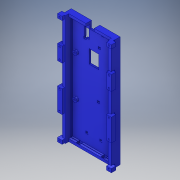
# Autodesk Inventor part: BODY_BOTTOM_2
Saved by Autodesk Inventor 2017 (Build 210142000, 142)
## iProperties
Created: 2018-07-28
Part Number: BODY_BOTTOM_2
Material: Generic
Document SubType Name: Modeling
Designer: Alexander Miller
Density: 1 g/cm^3
Appearance: Blue - Wall Paint - Glossy
Author: Alexander Miller
Autodesk Inventor part; units mm, degrees
ref_plane "YZ Plane" through (0, 0, 0) normal (1, 0, 0) x (0, 1, 0)
ref_plane "XZ Plane" through (0, 0, 0) normal (0, 1, 0) x (-1, 0, 0)
ref_plane "XY Plane" through (0, 0, 0) normal (0, 0, 1) x (1, 0, 0)
sketch "Sketch1" plane through (0, 0, 0) normal (0, 0, 1) x (1, 0, 0)
  line L0 (-34.885, -79.35) -> (34.885, -79.35)
  line L1 (34.885, -79.35) -> (34.885, 79.35)
  line L2 (34.885, 79.35) -> (-34.885, 79.35)
  line L3 (-34.885, 79.35) -> (-34.885, -79.35)
  point P0 (0, 0)
  point P1 (0, 79.35)
  point P2 (34.885, 0)
  point P3 (0, -79.35)
  dimension "d0" = 158.7
  dimension "d1" = 69.77
  constraints: 8 end point, 3 midpoint, 2 parallel, 1 horizontal, 1 horizontal alignment, 1 perpendicular, 1 vertical alignment
  measures "d0" distance of L0.end L1.end
  measures "d1" distance of L1.end L2.end
extrude "Extrusion1" add sketch "Sketch1" along normal blind 5
sketch "Sketch3" plane through (0, 0, 5) normal (0, 0, 1) x (1, 0, 0)
  line L0 (-34.885, 79.35) -> (-30.5, 79.35)
  line L1 (-30.5, 79.35) -> (-30.5, -79.35)
  line L2 (-30.5, -79.35) -> (-34.885, -79.35)
  line L3 (-34.885, -79.35) -> (-34.885, 79.35)
  line L4 (30.5, 79.35) -> (34.885, 79.35)
  line L5 (34.885, 79.35) -> (34.885, -79.35)
  line L6 (34.885, -79.35) -> (30.5, -79.35)
  line L7 (30.5, -79.35) -> (30.5, 79.35)
  line L8 (34.885, 79.35) -> (-34.885, 79.35) projected
  line L9 (-34.885, 79.35) -> (-34.885, -79.35) projected
  line L10 (-34.885, -79.35) -> (34.885, -79.35) projected
  line L11 (34.885, -79.35) -> (34.885, 79.35) projected
  point P0 (0, 0)
  dimension "d14" = 4.385
  constraints: 16 end point, 7 collinear, 4 parallel, 2 horizontal, 2 perpendicular
  measures "d14" distance of L0.start L0.end
extrude "Extrusion3" add sketch "Sketch3" along normal blind 7.74 contours L0 L1 L2 L3 | L4 L5 L6 L7
sketch "Sketch4" plane through (0, 0, 12.74) normal (0, 0, 1) x (1, 0, 0)
  line L0 (31.885, -74.1) -> (38.635, -74.1)
  line L1 (38.635, -74.1) -> (38.635, -79.35)
  line L2 (38.635, -79.35) -> (31.885, -79.35)
  line L3 (31.885, -79.35) -> (31.885, -74.1)
  line L4 (30.5, 79.35) -> (30.5, -79.35) projected
  line L5 (30.5, -79.35) -> (34.885, -79.35) projected
  line L6 (31.885, -37.15) -> (38.635, -37.15)
  line L7 (38.635, -37.15) -> (38.635, -42.4)
  line L8 (38.635, -42.4) -> (31.885, -42.4)
  line L9 (31.885, -42.4) -> (31.885, -37.15)
  line L10 (31.885, -10.35) -> (38.635, -10.35)
  line L11 (38.635, -10.35) -> (38.635, -15.6)
  line L12 (38.635, -15.6) -> (31.885, -15.6)
  line L13 (31.885, -15.6) -> (31.885, -10.35)
  line L14 (31.885, 26.6) -> (38.635, 26.6)
  line L15 (38.635, 26.6) -> (38.635, 21.35)
  line L16 (38.635, 21.35) -> (31.885, 21.35)
  line L17 (31.885, 21.35) -> (31.885, 26.6)
  line L18 (31.885, 42.4) -> (38.635, 42.4)
  line L19 (38.635, 42.4) -> (38.635, 37.15)
  line L20 (38.635, 37.15) -> (31.885, 37.15)
  line L21 (31.885, 37.15) -> (31.885, 42.4)
  line L22 (31.885, 79.35) -> (38.635, 79.35)
  line L23 (38.635, 79.35) -> (38.635, 74.1)
  line L24 (38.635, 74.1) -> (31.885, 74.1)
  line L25 (31.885, 74.1) -> (31.885, 79.35)
  line L26 (34.885, 79.35) -> (30.5, 79.35) projected
  line L27 (41.26, 21.35) -> (29.26, 21.35) construction
  line L28 (29.26, 21.35) -> (29.26, -10.35) construction
  line L29 (29.26, -10.35) -> (41.26, -10.35) construction
  line L30 (41.26, -10.35) -> (41.26, 21.35) construction
  circle A0 centre (35.26, 0) radius 6 construction
  line L31 (0, -111.09) -> (0, 111.09) projected
  line L32 (-31.885, -74.1) -> (-38.635, -74.1)
  line L33 (-38.635, -74.1) -> (-38.635, -79.35)
  line L34 (-38.635, -79.35) -> (-31.885, -79.35)
  line L35 (-31.885, -79.35) -> (-31.885, -74.1)
  line L36 (-30.5, -79.35) -> (-34.885, -79.35)
  line L37 (-31.885, -37.15) -> (-38.635, -37.15)
  line L38 (-38.635, -37.15) -> (-38.635, -42.4)
  line L39 (-38.635, -42.4) -> (-31.885, -42.4)
  line L40 (-31.885, -42.4) -> (-31.885, -37.15)
  line L41 (-31.885, -10.35) -> (-38.635, -10.35)
  line L42 (-38.635, -10.35) -> (-38.635, -15.6)
  line L43 (-38.635, -15.6) -> (-31.885, -15.6)
  line L44 (-31.885, -15.6) -> (-31.885, -10.35)
  line L45 (-31.885, 26.6) -> (-38.635, 26.6)
  line L46 (-38.635, 26.6) -> (-38.635, 21.35)
  line L47 (-38.635, 21.35) -> (-31.885, 21.35)
  line L48 (-31.885, 21.35) -> (-31.885, 26.6)
  line L49 (-31.885, 42.4) -> (-38.635, 42.4)
  line L50 (-38.635, 42.4) -> (-38.635, 37.15)
  line L51 (-38.635, 37.15) -> (-31.885, 37.15)
  line L52 (-31.885, 37.15) -> (-31.885, 42.4)
  line L53 (-31.885, 79.35) -> (-38.635, 79.35)
  line L54 (-38.635, 79.35) -> (-38.635, 74.1)
  line L55 (-38.635, 74.1) -> (-31.885, 74.1)
  line L56 (-31.885, 74.1) -> (-31.885, 79.35)
  line L57 (-34.885, 79.35) -> (-30.5, 79.35)
  line L58 (-41.26, 21.35) -> (-29.26, 21.35) construction
  line L59 (-29.26, -10.35) -> (-41.26, -10.35) construction
  line L60 (-41.26, -10.35) -> (-41.26, 21.35) construction
  circle A1 centre (-35.26, 0) radius 6 construction
  line L61 (29.26, 17) -> (41.26, 17) construction
  line L62 (41.26, 17) -> (41.26, -6) construction
  line L63 (41.26, -6) -> (29.26, -6) construction
  line L64 (29.26, -6) -> (29.26, 17) construction
  line L65 (-38.635, -37.15) -> (-31.885, -37.15)
  line L66 (-31.885, -37.15) -> (-31.885, -15.6)
  line L67 (-31.885, -15.6) -> (-38.635, -15.6)
  line L68 (-38.635, -15.6) -> (-38.635, -37.15)
  line L69 (31.885, -37.15) -> (38.635, -37.15)
  line L70 (38.635, -37.15) -> (38.635, -15.6)
  line L71 (38.635, -15.6) -> (31.885, -15.6)
  line L72 (31.885, -15.6) -> (31.885, -37.15)
  line L73 (-38.635, 26.6) -> (-31.885, 26.6)
  line L74 (-31.885, 26.6) -> (-31.885, 37.15)
  line L75 (-31.885, 37.15) -> (-38.635, 37.15)
  line L76 (-38.635, 37.15) -> (-38.635, 26.6)
  line L77 (31.885, 26.6) -> (38.635, 26.6)
  line L78 (38.635, 26.6) -> (38.635, 37.15)
  line L79 (38.635, 37.15) -> (31.885, 37.15)
  line L80 (31.885, 37.15) -> (31.885, 26.6)
  line L81 (-31.885, 74.1) -> (-30.5, 74.1)
  line L82 (-30.5, 74.1) -> (-30.5, 79.35)
  line L83 (-30.5, 79.35) -> (-31.885, 79.35)
  line L84 (-31.885, 79.35) -> (-31.885, 74.1)
  line L85 (-31.885, 42.4) -> (-30.5, 42.4)
  line L86 (-30.5, 42.4) -> (-30.5, 21.35)
  line L87 (-30.5, 21.35) -> (-31.885, 21.35)
  line L88 (-31.885, 21.35) -> (-31.885, 42.4)
  line L89 (-31.885, -10.35) -> (-30.5, -10.35)
  line L90 (-30.5, -10.35) -> (-30.5, -42.4)
  line L91 (-30.5, -42.4) -> (-31.885, -42.4)
  line L92 (-31.885, -42.4) -> (-31.885, -10.35)
  line L93 (-31.885, -74.1) -> (-30.5, -74.1)
  line L94 (-30.5, -74.1) -> (-30.5, -79.35)
  line L95 (-30.5, -79.35) -> (-31.885, -79.35)
  line L96 (-31.885, -79.35) -> (-31.885, -74.1)
  line L97 (30.5, 79.35) -> (31.885, 79.35)
  line L98 (31.885, 79.35) -> (31.885, 74.1)
  line L99 (31.885, 74.1) -> (30.5, 74.1)
  line L100 (30.5, 74.1) -> (30.5, 79.35)
  line L101 (30.5, 42.4) -> (31.885, 42.4)
  line L102 (31.885, 42.4) -> (31.885, 21.35)
  line L103 (31.885, 21.35) -> (30.5, 21.35)
  line L104 (30.5, 21.35) -> (30.5, 42.4)
  line L105 (30.5, -10.35) -> (31.885, -10.35)
  line L106 (31.885, -10.35) -> (31.885, -42.4)
  line L107 (31.885, -42.4) -> (30.5, -42.4)
  line L108 (30.5, -42.4) -> (30.5, -10.35)
  line L109 (30.5, -74.1) -> (31.885, -74.1)
  line L110 (31.885, -74.1) -> (31.885, -79.35)
  line L111 (31.885, -79.35) -> (30.5, -79.35)
  line L112 (30.5, -79.35) -> (30.5, -74.1)
  line L113 (-30.5, -79.35) -> (-30.5, 79.35) projected
  line L114 (-34.885, -79.35) -> (-30.5, -79.35) projected
  point P0 (0, 0)
  point P1 (35.26, 74.1)
  point P2 (35.26, 42.4)
  point P3 (35.26, 37.15)
  point P4 (35.26, 26.6)
  point P5 (35.26, 21.35)
  point P6 (35.26, -10.35)
  point P7 (35.26, -15.6)
  point P8 (35.26, -37.15)
  point P9 (35.26, -42.4)
  point P10 (35.26, -74.1)
  point P11 (35.26, 21.35)
  point P12 (-35.26, 74.1)
  point P13 (-35.26, 42.4)
  point P14 (-35.26, 37.15)
  point P15 (-35.26, 26.6)
  point P16 (-35.26, 21.35)
  point P17 (-35.26, -10.35)
  point P18 (-35.26, -15.6)
  point P19 (-35.26, -37.15)
  point P20 (-35.26, -42.4)
  point P21 (-35.26, -74.1)
  point P22 (-35.26, 21.35)
  point P23 (29.26, 5.5)
  point P24 (29.26, 5.5)
  dimension "d17" = 6.75
  dimension "d18" = 1.385
  dimension "d19" = 5.25
  dimension "d40" = 31.7
  dimension "d41" = 31.7
  dimension "d42" = 31.7
  dimension "d43" = 12
  dimension "d44" = 23
  constraints: 218 end point, 44 symmetric about line, 40 parallel, 34 collinear, 20 horizontal, 20 perpendicular, 13 midpoint, 10 equal length, 5 vertical alignment, 3 tangent, 2 centre point, 2 coincident, 1 horizontal alignment, 1 other
  measures "d17" distance of L0.start L0.end
  measures "d18" distance between parallel lines of L3 L4
  measures "d19" distance of L0.end L1.end
  measures "d40" distance between parallel lines of L0 L8
  measures "d41" distance between parallel lines of L10 L16
  measures "d42" distance between parallel lines of L18 L24
  measures "d43" distance of L27.start L27.end
  measures "d44" distance between parallel lines of L63 L61
extrude "Extrusion4" add sketch "Sketch4" along normal blind 3.5 and the other way blind 5 contours L0 L1 L2 L3 | L9 L6 L7 L8 | L10 L11 L12 L13 | L72 L12 L70 L6 | L17 L14 L15 L16 | L18 L19 L20 L21 | L80 L20 L78 L14 | L25 L22 L23 L24 | L35 L34 L33 L32 | L39 L38 L37 L40 | L44 L43 L42 L41 | L37 L68 L43 L66 | L47 L46 L45 L48 | L52 L51 L50 L49 | L45 L76 L51 L74 | L55 L54 L53 L56
sketch "Sketch7" plane through (0, 0, 7.74) normal (0, 0, -1) x (-1, 0, 0)
  line L0 (-33.085, -78.85) -> (-37.435, -78.85)
  line L1 (-37.435, -78.85) -> (-37.435, -74.5)
  line L2 (-37.435, -74.5) -> (-33.085, -74.5)
  line L3 (-33.085, -74.5) -> (-33.085, -78.85)
  line L4 (-38.635, -74.1) -> (-38.635, -79.35) projected
  line L5 (-31.885, -79.35) -> (-38.635, -79.35) projected
  line L6 (-33.085, -37.65) -> (-37.435, -37.65)
  line L7 (-37.435, -37.65) -> (-37.435, -42)
  line L8 (-37.435, -42) -> (-33.085, -42)
  line L9 (-33.085, -42) -> (-33.085, -37.65)
  line L10 (-33.085, -10.75) -> (-37.435, -10.75)
  line L11 (-37.435, -10.75) -> (-37.435, -15.1)
  line L12 (-37.435, -15.1) -> (-33.085, -15.1)
  line L13 (-33.085, -15.1) -> (-33.085, -10.75)
  line L14 (-33.085, 26.1) -> (-37.435, 26.1)
  line L15 (-37.435, 26.1) -> (-37.435, 21.75)
  line L16 (-37.435, 21.75) -> (-33.085, 21.75)
  line L17 (-33.085, 21.75) -> (-33.085, 26.1)
  line L18 (-33.085, 42) -> (-37.435, 42)
  line L19 (-37.435, 42) -> (-37.435, 37.65)
  line L20 (-37.435, 37.65) -> (-33.085, 37.65)
  line L21 (-33.085, 37.65) -> (-33.085, 42)
  line L22 (-33.085, 78.85) -> (-37.435, 78.85)
  line L23 (-37.435, 78.85) -> (-37.435, 74.5)
  line L24 (-37.435, 74.5) -> (-33.085, 74.5)
  line L25 (-33.085, 74.5) -> (-33.085, 78.85)
  line L26 (-38.635, 79.35) -> (-38.635, 74.1) projected
  line L27 (0, -111.09) -> (0, 111.09) projected
  line L28 (33.085, -78.85) -> (37.435, -78.85)
  line L29 (37.435, -78.85) -> (37.435, -74.5)
  line L30 (37.435, -74.5) -> (33.085, -74.5)
  line L31 (33.085, -74.5) -> (33.085, -78.85)
  line L32 (33.085, -37.65) -> (37.435, -37.65)
  line L33 (37.435, -37.65) -> (37.435, -42)
  line L34 (37.435, -42) -> (33.085, -42)
  line L35 (33.085, -42) -> (33.085, -37.65)
  line L36 (33.085, -10.75) -> (37.435, -10.75)
  line L37 (37.435, -10.75) -> (37.435, -15.1)
  line L38 (37.435, -15.1) -> (33.085, -15.1)
  line L39 (33.085, -15.1) -> (33.085, -10.75)
  line L40 (33.085, 26.1) -> (37.435, 26.1)
  line L41 (37.435, 26.1) -> (37.435, 21.75)
  line L42 (37.435, 21.75) -> (33.085, 21.75)
  line L43 (33.085, 21.75) -> (33.085, 26.1)
  line L44 (33.085, 42) -> (37.435, 42)
  line L45 (37.435, 42) -> (37.435, 37.65)
  line L46 (37.435, 37.65) -> (33.085, 37.65)
  line L47 (33.085, 37.65) -> (33.085, 42)
  line L48 (33.085, 78.85) -> (37.435, 78.85)
  line L49 (37.435, 78.85) -> (37.435, 74.5)
  line L50 (37.435, 74.5) -> (33.085, 74.5)
  line L51 (33.085, 74.5) -> (33.085, 78.85)
  line L52 (-38.635, -79.35) -> (-34.885, -79.35) projected
  line L53 (-34.885, -74.1) -> (-34.885, -79.35) projected
  line L54 (-38.635, -79.35) -> (-34.885, -79.35)
  line L55 (-34.885, -79.35) -> (-34.885, -74.1)
  line L56 (-34.885, -74.1) -> (-38.635, -74.1)
  line L57 (-38.635, -74.1) -> (-38.635, -79.35)
  line L58 (-34.885, 79.35) -> (-38.635, 79.35) projected
  line L59 (-38.635, -42.4) -> (-34.885, -42.4) projected
  line L60 (-34.885, -10.35) -> (-38.635, -10.35) projected
  line L61 (-38.635, 21.35) -> (-34.885, 21.35) projected
  line L62 (-34.885, 42.4) -> (-38.635, 42.4) projected
  line L63 (-38.635, -42.4) -> (-34.885, -42.4)
  line L64 (-34.885, -42.4) -> (-34.885, -10.35)
  line L65 (-34.885, -10.35) -> (-38.635, -10.35)
  line L66 (-38.635, -10.35) -> (-38.635, -42.4)
  line L67 (-38.635, 21.35) -> (-38.635, 42.4) projected
  line L68 (-38.635, 21.35) -> (-34.885, 21.35)
  line L69 (-34.885, 21.35) -> (-34.885, 42.4)
  line L70 (-34.885, 42.4) -> (-38.635, 42.4)
  line L71 (-38.635, 42.4) -> (-38.635, 21.35)
  line L72 (-31.885, 74.1) -> (-38.635, 74.1) projected
  line L73 (-34.885, -79.35) -> (-34.885, 79.35) projected
  line L74 (-38.635, 74.1) -> (-34.885, 74.1)
  line L75 (-34.885, 74.1) -> (-34.885, 79.35)
  line L76 (-34.885, 79.35) -> (-38.635, 79.35)
  line L77 (-38.635, 79.35) -> (-38.635, 74.1)
  line L78 (38.635, -74.1) -> (38.635, -79.35) projected
  line L79 (34.885, 79.35) -> (34.885, -79.35) projected
  line L80 (38.635, -74.1) -> (34.885, -74.1)
  line L81 (34.885, -74.1) -> (34.885, -79.35)
  line L82 (34.885, -79.35) -> (38.635, -79.35)
  line L83 (38.635, -79.35) -> (38.635, -74.1)
  line L84 (38.635, -42.4) -> (38.635, -10.35) projected
  line L85 (34.885, -42.4) -> (34.885, -10.35) projected
  line L86 (38.635, -10.35) -> (34.885, -10.35)
  line L87 (34.885, -10.35) -> (34.885, -42.4)
  line L88 (34.885, -42.4) -> (38.635, -42.4)
  line L89 (38.635, -42.4) -> (38.635, -10.35)
  line L90 (38.635, 21.35) -> (38.635, 42.4) projected
  line L91 (38.635, 42.4) -> (34.885, 42.4)
  line L92 (34.885, 42.4) -> (34.885, 21.35)
  line L93 (34.885, 21.35) -> (38.635, 21.35)
  line L94 (38.635, 21.35) -> (38.635, 42.4)
  line L95 (38.635, 79.35) -> (38.635, 74.1) projected
  line L96 (38.635, 79.35) -> (34.885, 79.35)
  line L97 (34.885, 79.35) -> (34.885, 74.1)
  line L98 (34.885, 74.1) -> (38.635, 74.1)
  line L99 (38.635, 74.1) -> (38.635, 79.35)
  point P0 (0, 0)
  point P1 (-37.435, -76.675)
  point P2 (-35.26, -79.35)
  point P3 (-35.26, -78.85)
  point P4 (-35.26, -74.5)
  point P5 (-35.26, -42)
  point P6 (-35.26, -37.65)
  point P7 (-35.26, -15.1)
  point P8 (-35.26, -10.75)
  point P9 (-35.26, 21.75)
  point P10 (-35.26, 26.1)
  point P11 (-35.26, 37.65)
  point P12 (-35.26, 42)
  point P13 (-35.26, 74.5)
  point P14 (-37.435, -39.825)
  point P15 (-38.635, -39.825)
  point P16 (-37.435, -12.925)
  point P17 (-38.635, -12.925)
  point P18 (-37.435, 23.925)
  point P19 (-38.635, 23.925)
  point P20 (-37.435, 39.825)
  point P21 (-38.635, 39.825)
  point P22 (-37.435, 76.675)
  point P23 (-38.635, 76.725)
  point P24 (37.435, -76.675)
  point P25 (31.885, -79.35)
  point P26 (35.26, -79.35)
  point P27 (35.26, -78.85)
  point P28 (35.26, -74.5)
  point P29 (35.26, -42)
  point P30 (35.26, -37.65)
  point P31 (35.26, -15.1)
  point P32 (35.26, -10.75)
  point P33 (35.26, 21.75)
  point P34 (35.26, 26.1)
  point P35 (35.26, 37.65)
  point P36 (35.26, 42)
  point P37 (35.26, 74.5)
  point P38 (37.435, -39.825)
  point P39 (37.435, -12.925)
  point P40 (37.435, 23.925)
  point P41 (37.435, 39.825)
  point P42 (37.435, 76.725)
  dimension "d45" = 4.35
  dimension "d142" = 2.675
  dimension "d143" = 2.675
  dimension "d144" = 2.575
  dimension "d145" = 2.575
  dimension "d146" = 2.575
  dimension "d147" = 2.575
  constraints: 160 end point, 42 symmetric about line, 28 parallel, 19 midpoint, 14 horizontal, 14 perpendicular, 11 equal length, 6 vertical alignment, 4 horizontal alignment, 4 point on line
  measures "d45" distance of L0.end L1.end
  measures "d142" distance from line of point (-37.435, -76.675) L5
  measures "d143" distance from line of point (-37.435, 76.675) L58
  measures "d144" distance from line of L59 point (-37.435, -39.825)
  measures "d145" distance from line of point (-37.435, -12.925) L60
  measures "d146" distance from line of L61 point (-37.435, 23.925)
  measures "d147" distance from line of point (-37.435, 39.825) L62
extrude "Extrusion7" cut sketch "Sketch7" against normal blind 2.075
sketch "Sketch8" plane through (0, 0, 16.24) normal (0, 0, 1) x (1, 0, 0)
  circle A0 centre (35.26, -76.675) radius 1.175
  line L0 (31.885, -74.1) -> (31.885, -79.35) projected
  line L1 (38.635, -74.1) -> (31.885, -74.1) projected
  circle A1 centre (35.26, -39.825) radius 1.175
  circle A2 centre (35.26, -12.925) radius 1.175
  circle A3 centre (35.26, 23.925) radius 1.175
  circle A4 centre (35.26, 39.825) radius 1.175
  circle A5 centre (35.26, 76.675) radius 1.175
  line L2 (31.885, 79.35) -> (31.885, 74.1) projected
  line L3 (0, -111.09) -> (0, 111.09) projected
  circle A6 centre (-35.26, -76.675) radius 1.175
  circle A7 centre (-35.26, -39.825) radius 1.175
  circle A8 centre (-35.26, -12.925) radius 1.175
  circle A9 centre (-35.26, 23.925) radius 1.175
  circle A10 centre (-35.26, 39.825) radius 1.175
  circle A11 centre (-35.26, 76.675) radius 1.175
  line L4 (31.885, -79.35) -> (38.635, -79.35) projected
  line L5 (31.885, -42.4) -> (38.635, -42.4) projected
  line L6 (38.635, -10.35) -> (31.885, -10.35) projected
  line L7 (31.885, 21.35) -> (38.635, 21.35) projected
  line L8 (38.635, 42.4) -> (31.885, 42.4) projected
  line L9 (38.635, 79.35) -> (31.885, 79.35) projected
  point P0 (0, 0)
  point P1 (31.885, -76.725)
  point P2 (35.26, -74.1)
  point P3 (31.885, 76.725)
  point P4 (31.885, 39.825)
  point P5 (31.885, 23.925)
  point P6 (31.885, -12.925)
  point P7 (31.885, -39.825)
  point P8 (-35.26, -74.1)
  point P9 (-38.635, -74.1)
  dimension "d48" = 2.35
  dimension "d148" = 2.675
  dimension "d149" = 2.575
  dimension "d150" = 2.575
  dimension "d151" = 2.575
  dimension "d152" = 2.575
  dimension "d153" = 2.675
  constraints: 12 centre point, 8 symmetric about line, 6 vertical alignment, 5 equal radius, 4 horizontal alignment, 3 midpoint, 6 other
  measures "d48" diameter of A0
  measures "d148" distance from line of L4 A0.centre
  measures "d149" distance from line of L5 A1.centre
  measures "d150" distance from line of L6 A2.centre
  measures "d151" distance from line of L7 A3.centre
  measures "d152" distance from line of A4.centre L8
  measures "d153" distance from line of L9 A5.centre
extrude "Extrusion8" cut sketch "Sketch8" against normal up to surface (6.425 mm away)
sketch "Sketch9" plane through (0, 0, 5) normal (0, 0, 1) x (1, 0, 0)
  circle A0 centre (-25, 31.875) radius 1.25
  line L0 (30.5, 79.35) -> (-30.5, 79.35) projected
  line L1 (0, -111.09) -> (0, 111.09) projected
  line L2 (-48.839, 0) -> (48.839, 0) projected
  circle A1 centre (-25, -26.375) radius 1.25
  circle A2 centre (25, 31.875) radius 1.25
  circle A3 centre (25, -26.375) radius 1.25
  point P0 (0, 0)
  dimension "d52" = 31.875
  dimension "d53" = 25
  dimension "d54" = 2.5
  dimension "d57" = 58.25
  constraints: 4 centre point, 2 symmetric about line, 1 equal radius, 1 vertical alignment, 2 other
  measures "d52" vertical distance of point (0, 0) A0.centre
  measures "d53" horizontal distance of A0.centre point (0, 0)
  measures "d54" diameter of A0
  measures "d57" distance of A1.centre A0.centre
extrude "Extrusion9" cut sketch "Sketch9" against normal through all
sketch "Sketch10" plane through (0, 0, 5) normal (0, 0, 1) x (1, 0, 0)
  line L0 (30.25, -75.25) -> (-30.25, -75.25)
  line L1 (-30.25, -75.25) -> (-30.25, 75.25)
  line L2 (-30.25, 75.25) -> (30.25, 75.25)
  line L3 (30.25, 75.25) -> (30.25, -75.25)
  circle A0 centre (25, -26.375) radius 3.25
  circle A1 centre (-25, -26.375) radius 3.25
  circle A2 centre (25, 31.875) radius 3.25
  circle A3 centre (-25, 31.875) radius 3.25
  circle A4 centre (25, -26.375) radius 1.25 projected
  circle A5 centre (-25, -26.375) radius 1.25 projected
  circle A6 centre (-25, 31.875) radius 1.25 projected
  circle A7 centre (25, 31.875) radius 1.25 projected
  point P0 (0, 0)
  point P1 (-30.25, 0)
  point P2 (0, -75.25)
  dimension "d58" = 150.5
  dimension "d59" = 60.5
  dimension "d61" = 2
  constraints: 8 end point, 4 centre point, 4 concentric, 3 equal radius, 2 midpoint, 2 parallel, 1 horizontal, 1 horizontal alignment, 1 perpendicular, 1 vertical alignment
  measures "d58" distance of L0.end L1.end
  measures "d59" distance of L0.start L0.end
  measures "d61" radial gap between concentric circles of A0 A4
extrude "Extrusion10" cut sketch "Sketch10" against normal blind 2.5 contours L0 L1 L2 L3
sketch "Sketch12" plane through (0, 0, 5) normal (0, 0, 1) x (1, 0, 0)
  line L0 (-6, 79.35) -> (6, 79.35)
  line L1 (6, 79.35) -> (6, 70)
  line L2 (6, 70) -> (-6, 70)
  line L3 (-6, 70) -> (-6, 79.35)
  line L4 (30.5, 79.35) -> (-30.5, 79.35) projected
  point P0 (0, 0)
  point P1 (0, 79.35)
  point P2 (0, 79.35)
  dimension "d68" = 9.35
  dimension "d69" = 12
  constraints: 8 end point, 2 midpoint, 2 parallel, 1 coincident, 1 collinear, 1 horizontal, 1 perpendicular
  measures "d68" distance of L2.end L0.start
  measures "d69" distance of L1.end L2.end
extrude "Extrusion12" cut sketch "Sketch12" against normal through all
sketch "Sketch13" plane through (0, 0, 0) normal (0, 0, -1) x (-1, 0, 0)
  line L0 (-7, 45.14) -> (7, 45.14)
  line L1 (7, 45.14) -> (7, 38.54)
  line L2 (7, 38.54) -> (-7, 38.54)
  line L3 (-7, 38.54) -> (-7, 45.14)
  line L4 (-7, 38.79) -> (7, 38.79)
  line L5 (7, 38.79) -> (7, 32.19)
  line L6 (7, 32.19) -> (-7, 32.19)
  line L7 (-7, 32.19) -> (-7, 38.79)
  line L8 (-7, 32.44) -> (7, 32.44)
  line L9 (7, 32.44) -> (7, 25.84)
  line L10 (7, 25.84) -> (-7, 25.84)
  line L11 (-7, 25.84) -> (-7, 32.44)
  line L12 (-13.791, 74.201) -> (-10.791, 74.201)
  line L13 (-10.791, 74.201) -> (-10.791, 71.201)
  line L14 (-10.791, 71.201) -> (-13.791, 71.201)
  line L15 (-13.791, 71.201) -> (-13.791, 74.201)
  line L16 (-9.244, 54.465) -> (-6.244, 54.465)
  line L17 (-6.244, 54.465) -> (-6.244, 51.465)
  line L18 (-6.244, 51.465) -> (-9.244, 51.465)
  line L19 (-9.244, 51.465) -> (-9.244, 54.465)
  line L20 (11.279, 56.853) -> (14.279, 56.853)
  line L21 (14.279, 56.853) -> (14.279, 53.853)
  line L22 (14.279, 53.853) -> (11.279, 53.853)
  line L23 (11.279, 53.853) -> (11.279, 56.853)
  line L24 (-8.051, -13.023) -> (-5.051, -13.023)
  line L25 (-5.051, -13.023) -> (-5.051, -16.023)
  line L26 (-5.051, -16.023) -> (-8.051, -16.023)
  line L27 (-8.051, -16.023) -> (-8.051, -13.023)
  line L28 (-11.53, -59.149) -> (-8.53, -59.149)
  line L29 (-8.53, -59.149) -> (-8.53, -62.149)
  line L30 (-8.53, -62.149) -> (-11.53, -62.149)
  line L31 (-11.53, -62.149) -> (-11.53, -59.149)
  line L32 (8.485, -59.149) -> (11.485, -59.149)
  line L33 (11.485, -59.149) -> (11.485, -62.149)
  line L34 (11.485, -62.149) -> (8.485, -62.149)
  line L35 (8.485, -62.149) -> (8.485, -59.149)
  line L36 (-13.791, 72.296) -> (-10.791, 72.296)
  line L37 (-10.791, 72.296) -> (-10.791, 69.296)
  line L38 (-10.791, 69.296) -> (-13.791, 69.296)
  line L39 (-13.791, 69.296) -> (-13.791, 72.296)
  line L40 (6.637, 69.673) -> (13.637, 69.673)
  line L41 (13.637, 69.673) -> (13.637, 62.673)
  line L42 (13.637, 62.673) -> (6.637, 62.673)
  line L43 (6.637, 62.673) -> (6.637, 69.673)
  line L44 (13.637, 63.399) -> (6.637, 63.399)
  line L45 (6.637, 63.399) -> (6.637, 56.399)
  line L46 (6.637, 56.399) -> (13.637, 56.399)
  line L47 (13.637, 56.399) -> (13.637, 63.399)
  point P0 (0, 0)
  point P1 (0, 38.54)
  point P2 (7, 41.84)
  point P3 (0, 38.79)
  point P4 (0, 32.19)
  point P5 (0, 32.44)
  point P6 (7, 35.49)
  point P7 (7, 29.14)
  point P8 (-10.791, 72.701)
  point P9 (-12.291, 71.201)
  point P10 (-12.291, 72.296)
  point P11 (-10.791, 70.796)
  point P12 (-6.244, 52.965)
  point P13 (-7.744, 51.465)
  point P14 (12.779, 53.853)
  point P15 (11.279, 55.353)
  point P16 (-6.551, -13.023)
  point P17 (-5.051, -14.523)
  point P18 (-10.03, -59.149)
  point P19 (-11.53, -60.649)
  point P20 (9.985, -59.149)
  point P21 (11.485, -60.649)
  point P22 (13.637, 66.173)
  point P23 (10.137, 62.673)
  point P24 (6.637, 59.899)
  point P25 (10.137, 56.399)
  point P26 (10.137, 63.399)
  dimension "d72" = 41.84
  dimension "d73" = 14
  dimension "d74" = 6.6
  dimension "d77" = 35.49
  dimension "d78" = 29.14
  dimension "d79" = 12.291
  dimension "d80" = 72.701
  dimension "d81" = 3
  dimension "d83" = 70.796
  dimension "d84" = 7.744
  dimension "d85" = 52.965
  dimension "d86" = 12.779
  dimension "d87" = 55.353
  dimension "d88" = 6.551
  dimension "d89" = 14.523
  dimension "d90" = 10.03
  dimension "d91" = 60.649
  dimension "d92" = 9.985
  dimension "d93" = 60.649
  dimension "d133" = 10.137
  dimension "d134" = 66.173
  dimension "d135" = 7
  dimension "d136" = 7
  dimension "d138" = 59.899
  constraints: 96 end point, 26 midpoint, 24 parallel, 19 equal length, 12 horizontal, 12 perpendicular, 5 vertical alignment
  measures "d72" vertical distance of point (7, 41.84) point (0, 0)
  measures "d73" distance of L0.start L0.end
  measures "d74" distance of L2.end L0.start
  measures "d77" vertical distance of point (7, 35.49) point (0, 0)
  measures "d78" vertical distance of point (7, 29.14) point (0, 0)
  measures "d79" horizontal distance of point (-12.291, 71.201) point (0, 0)
  measures "d80" vertical distance of point (0, 0) point (-10.791, 72.701)
  measures "d81" distance of L14.end L12.start
  measures "d83" vertical distance of point (0, 0) point (-10.791, 70.796)
  measures "d84" horizontal distance of point (-7.744, 51.465) point (0, 0)
  measures "d85" vertical distance of point (-6.244, 52.965) point (0, 0)
  measures "d86" horizontal distance of point (0, 0) point (12.779, 53.853)
  measures "d87" vertical distance of point (0, 0) point (11.279, 55.353)
  measures "d88" horizontal distance of point (-6.551, -13.023) point (0, 0)
  measures "d89" vertical distance of point (-5.051, -14.523) point (0, 0)
  measures "d90" horizontal distance of point (-10.03, -59.149) point (0, 0)
  measures "d91" vertical distance of point (0, 0) point (-11.53, -60.649)
  measures "d92" horizontal distance of point (9.985, -59.149) point (0, 0)
  measures "d93" vertical distance of point (11.485, -60.649) point (0, 0)
  measures "d133" horizontal distance of point (10.137, 62.673) point (0, 0)
  measures "d134" vertical distance of point (0, 0) point (13.637, 66.173)
  measures "d135" distance of L40.start L40.end
  measures "d136" distance of L44.start L44.end
  measures "d138" vertical distance of point (6.637, 59.899) point (0, 0)
extrude "Extrusion13" cut sketch "Sketch13" against normal through all
sketch "Sketch14" plane through (0, 0, 0) normal (0, 0, -1) x (-1, 0, 0)
  line L0 (-27.175, 34.05) -> (-22.825, 34.05)
  line L1 (-22.825, 34.05) -> (-22.825, 29.7)
  line L2 (-22.825, 29.7) -> (-27.175, 29.7)
  line L3 (-27.175, 29.7) -> (-27.175, 34.05)
  line L4 (22.825, 34.05) -> (27.175, 34.05)
  line L5 (27.175, 34.05) -> (27.175, 29.7)
  line L6 (27.175, 29.7) -> (22.825, 29.7)
  line L7 (22.825, 29.7) -> (22.825, 34.05)
  line L8 (22.825, -24.2) -> (27.175, -24.2)
  line L9 (27.175, -24.2) -> (27.175, -28.55)
  line L10 (27.175, -28.55) -> (22.825, -28.55)
  line L11 (22.825, -28.55) -> (22.825, -24.2)
  line L12 (-27.175, -24.2) -> (-22.825, -24.2)
  line L13 (-22.825, -24.2) -> (-22.825, -28.55)
  line L14 (-22.825, -28.55) -> (-27.175, -28.55)
  line L15 (-27.175, -28.55) -> (-27.175, -24.2)
  circle A0 centre (-25, 31.875) radius 1.25 projected
  circle A1 centre (25, 31.875) radius 1.25 projected
  line L16 (-7, 25.84) -> (-7, 45.14) projected
  line L17 (-7, 45.14) -> (7, 45.14) projected
  line L18 (7, 45.14) -> (7, 25.84) projected
  line L19 (7, 25.84) -> (-7, 25.84) projected
  line L20 (-10.791, 74.201) -> (-10.791, 69.296) projected
  line L21 (-10.791, 69.296) -> (-13.791, 69.296) projected
  line L22 (-13.791, 69.296) -> (-13.791, 74.201) projected
  line L23 (-13.791, 74.201) -> (-10.791, 74.201) projected
  line L24 (-11.53, -62.149) -> (-11.53, -59.149) projected
  line L25 (-11.53, -59.149) -> (-8.53, -59.149) projected
  line L26 (-8.53, -59.149) -> (-8.53, -62.149) projected
  line L27 (-8.53, -62.149) -> (-11.53, -62.149) projected
  line L28 (11.279, 53.853) -> (11.279, 56.399) projected
  line L29 (13.637, 56.853) -> (14.279, 56.853) projected
  line L30 (14.279, 56.853) -> (14.279, 53.853) projected
  line L31 (14.279, 53.853) -> (11.279, 53.853) projected
  line L32 (-9.244, 51.465) -> (-9.244, 54.465) projected
  line L33 (-9.244, 54.465) -> (-6.244, 54.465) projected
  line L34 (-6.244, 54.465) -> (-6.244, 51.465) projected
  line L35 (-6.244, 51.465) -> (-9.244, 51.465) projected
  line L36 (-8.051, -16.023) -> (-8.051, -13.023) projected
  line L37 (-8.051, -13.023) -> (-5.051, -13.023) projected
  line L38 (-5.051, -13.023) -> (-5.051, -16.023) projected
  line L39 (-5.051, -16.023) -> (-8.051, -16.023) projected
  line L40 (8.485, -62.149) -> (8.485, -59.149) projected
  line L41 (8.485, -59.149) -> (11.485, -59.149) projected
  line L42 (11.485, -59.149) -> (11.485, -62.149) projected
  line L43 (11.485, -62.149) -> (8.485, -62.149) projected
  line L44 (6, 79.35) -> (6, 70) projected
  line L45 (6, 70) -> (-6, 70) projected
  line L46 (-6, 70) -> (-6, 79.35) projected
  line L47 (-34.885, 79.35) -> (-6, 79.35) projected
  line L48 (-34.885, -79.35) -> (-34.885, 79.35) projected
  line L49 (34.885, -79.35) -> (-34.885, -79.35) projected
  line L50 (34.885, 79.35) -> (34.885, -79.35) projected
  circle A2 centre (-25, 31.875) radius 1.25 projected
  circle A3 centre (25, -26.375) radius 1.25 projected
  circle A4 centre (25, 31.875) radius 1.25 projected
  circle A5 centre (-25, -26.375) radius 1.25 projected
  circle A6 centre (25, -26.375) radius 1.25 projected
  line L51 (6, 79.35) -> (34.885, 79.35) projected
  line L52 (13.637, 69.673) -> (13.637, 56.853) projected
  line L53 (11.279, 56.399) -> (6.637, 56.399) projected
  line L54 (6.637, 56.399) -> (6.637, 69.673) projected
  line L55 (6.637, 69.673) -> (13.637, 69.673) projected
  point P0 (0, 0)
  point P1 (-22.825, 31.875)
  point P2 (22.825, 31.875)
  point P3 (22.825, -26.375)
  point P4 (-22.825, -26.375)
  point P5 (-25, 34.05)
  point P6 (25, 34.05)
  point P7 (25, -24.2)
  point P8 (-25, -24.2)
  dimension "d94" = 4.35
  constraints: 32 end point, 8 midpoint, 8 parallel, 7 equal length, 4 horizontal, 4 horizontal alignment, 4 perpendicular, 4 vertical alignment
  measures "d94" distance of L0.start L0.end
extrude "Extrusion14" cut sketch "Sketch14" against normal blind 2.15 contours L0 L1 L2 L3 | L4 L5 L6 L7 | L8 L9 L10 L11 | L12 L13 L14 L15
sketch "Sketch16" plane through (0, 0, 5) normal (0, 0, 1) x (1, 0, 0)
  line L0 (-30.5, 79.35) -> (-6, 79.35)
  line L1 (-6, 79.35) -> (-6, 75.6)
  line L2 (-6, 75.6) -> (-30.5, 75.6)
  line L3 (-30.5, 75.6) -> (-30.5, 79.35)
  line L4 (6, 79.35) -> (30.5, 79.35)
  line L5 (30.5, 79.35) -> (30.5, 75.6)
  line L6 (30.5, 75.6) -> (6, 75.6)
  line L7 (6, 75.6) -> (6, 79.35)
  line L8 (-30.5, -75.6) -> (30.5, -75.6)
  line L9 (30.5, -75.6) -> (30.5, -79.35)
  line L10 (30.5, -79.35) -> (-30.5, -79.35)
  line L11 (-30.5, -79.35) -> (-30.5, -75.6)
  line L12 (-30.5, 79.35) -> (-30.5, -79.35) projected
  line L13 (-6, 79.35) -> (-30.5, 79.35) projected
  line L14 (30.5, 79.35) -> (6, 79.35) projected
  line L15 (6, 79.35) -> (6, 75.25) projected
  line L16 (30.5, -79.35) -> (30.5, 79.35) projected
  line L17 (-30.5, -79.35) -> (30.5, -79.35) projected
  line L18 (-6, 75.25) -> (-6, 79.35) projected
  line L19 (-30.25, 75.25) -> (-6, 75.25) projected
  line L20 (30.25, -75.25) -> (-30.25, -75.25) projected
  point P0 (0, 0)
  dimension "d110" = 0.35
  dimension "d111" = 0.35
  constraints: 24 end point, 10 collinear, 6 parallel, 3 horizontal, 3 perpendicular
  measures "d110" distance between parallel lines of L19 L2
  measures "d111" distance between parallel lines of L8 L20
extrude "Extrusion15" add sketch "Sketch16" along normal blind 3
sketch "Sketch17" plane through (-30.25, -75.25, 5) normal (0, 1, 0) x (1, 0, 0)
  line L0 (9.9, 2.85) -> (15.25, 2.85)
  line L1 (15.25, 2.85) -> (15.25, -2.5)
  line L2 (15.25, -2.5) -> (9.9, -2.5)
  line L3 (9.9, -2.5) -> (9.9, 2.85)
  line L4 (45.25, 2.85) -> (50.6, 2.85)
  line L5 (50.6, 2.85) -> (50.6, -2.5)
  line L6 (50.6, -2.5) -> (45.25, -2.5)
  line L7 (45.25, -2.5) -> (45.25, 2.85)
  line L8 (45.25, 0.175) -> (15.25, 0.175) construction
  line L9 (60.5, 0) -> (0, 0) construction
  line L10 (60.75, -3) -> (-0.25, -3) construction
  point P0 (30.25, 5)
  point P1 (30.25, 0.175)
  point P2 (30.25, 0)
  dimension "d114" = 30
  dimension "d115" = 0.5
  dimension "d116" = 5.35
  constraints: 18 end point, 4 midpoint, 4 parallel, 3 equal length, 3 perpendicular, 2 horizontal, 1 horizontal alignment, 1 vertical alignment
  measures "d114" distance of L8.start L8.end
  measures "d115" distance between parallel lines of L6 L10
  measures "d116" distance of L5.end L6.end
extrude "Extrusion16" cut sketch "Sketch17" against normal blind 3.7
sketch "Sketch18" plane through (-30.25, 75.25, 2.5) normal (0, -1, 0) x (1, 0, 0)
  line L0 (15.25, -0.35) -> (9.9, -0.35)
  line L1 (9.9, -0.35) -> (9.9, 5)
  line L2 (9.9, 5) -> (15.25, 5)
  line L3 (15.25, 5) -> (15.25, -0.35)
  line L4 (50.6, -0.35) -> (45.25, -0.35)
  line L5 (45.25, -0.35) -> (45.25, 5)
  line L6 (45.25, 5) -> (50.6, 5)
  line L7 (50.6, 5) -> (50.6, -0.35)
  line L8 (15.25, 2.325) -> (45.25, 2.325) construction
  line L9 (-0.25, 5.5) -> (24.25, 5.5) projected
  point P0 (30.25, -2.5)
  point P1 (30.25, 2.325)
  dimension "d119" = 30
  dimension "d120" = 5.35
  dimension "d121" = 0.5
  constraints: 18 end point, 4 parallel, 3 equal length, 3 midpoint, 3 perpendicular, 2 horizontal, 1 horizontal alignment, 1 vertical alignment
  measures "d119" distance of L8.start L8.end
  measures "d120" distance of L1.end L2.end
  measures "d121" distance between parallel lines of L2 L9
extrude "Extrusion17" cut sketch "Sketch18" against normal blind 3.7
chamfer "Chamfer6" distance 0.5 angle 45 12 edges at (-34.885, 76.675, 7.74) (-34.885, 39.825, 7.74) (-34.885, 23.925, 7.74) (-34.885, -12.925, 7.74) (-34.885, -39.825, 7.74) (-34.885, -76.675, 7.74) (34.885, 76.675, 7.74) (34.885, 39.825, 7.74) (34.885, 23.925, 7.74) (34.885, -12.925, 7.74) (34.885, -39.825, 7.74) (34.885, -76.675, 7.74)
equation "\"d15\" = offset_z"
equation "\"d41\" = d40"
equation "\"d42\" = d40"
equation "\"d43\" = servo_B"
equation "\"d44\" = servo_A"
equation "\"d45\" = nut_A"
equation "\"d46\" = nut_B + Tolerance"
equation "\"d49\" = nut_B + Tolerance"
equation "\"d55\" = nut_B + Tolerance"
equation "\"d95\" = nut_B_1"
equation "\"offset_x\" = 4.885"
equation "\"offset_y\" = -1"
equation "\"offset_z\" = 7.74"
equation "\"servo_B\" = 12"
equation "\"servo_A\" = 23"
equation "\"nut_A\" = 4.35"
equation "\"nut_B\" = 1.725"
equation "\"Tolerance\" = 0.35"
equation "\"nut_B_1\" = 2.15"
body "Solid1"
